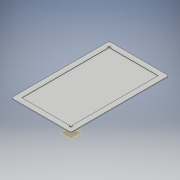
# Autodesk Inventor part: Lid
Saved by Autodesk Inventor 2019 (Build 230136000, 136)
## iProperties
Created: 2018-10-23
Part Number: Lid
Material: Generic
Document SubType Name: Modeling
Designer: Administrator
Density: 1 g/cm^3
Appearance: Default
Author: Administrator
Autodesk Inventor part; units mm, degrees
ref_plane "YZ Plane" through (0, 0, 0) normal (1, 0, 0) x (0, 1, 0)
ref_plane "XZ Plane" through (0, 0, 0) normal (0, 1, 0) x (-1, 0, 0)
ref_plane "XY Plane" through (0, 0, 0) normal (0, 0, 1) x (1, 0, 0)
ref_plane "Work Plane1" through (0, 41.656, 0) normal (0, 1, 0) x (1, 0, 0)
sketch "Sketch2" plane through (0, 41.656, 0) normal (0, 1, 0) x (1, 0, 0)
  line L0 (-118.364, 207.264) -> (-10.414, 207.264) projected
  arc A0 (-4.064, 200.914) -> (-10.414, 207.264) centre (-10.414, 200.914) ccw projected
  line L1 (-4.064, 200.914) -> (-4.064, 10.414) projected
  arc A1 (-10.414, 4.064) -> (-4.064, 10.414) centre (-10.414, 10.414) ccw projected
  line L2 (-10.414, 4.064) -> (-118.364, 4.064) projected
  arc A2 (-124.714, 10.414) -> (-118.364, 4.064) centre (-118.364, 10.414) ccw projected
  line L3 (-124.714, 10.414) -> (-124.714, 200.914) projected
  arc A3 (-118.364, 207.264) -> (-124.714, 200.914) centre (-118.364, 200.914) ccw projected
  line L4 (-128.778, 208.153) -> (-128.778, 3.175) projected
  arc A4 (-128.778, 3.175) -> (-125.603, 0) centre (-125.603, 3.175) ccw projected
  line L5 (-125.603, 0) -> (-3.175, 0) projected
  arc A5 (-3.175, 0) -> (0, 3.175) centre (-3.175, 3.175) ccw projected
  line L6 (0, 3.175) -> (0, 208.153) projected
  arc A6 (0, 208.153) -> (-3.175, 211.328) centre (-3.175, 208.153) ccw projected
  line L7 (-3.175, 211.328) -> (-125.603, 211.328) projected
  arc A7 (-125.603, 211.328) -> (-128.778, 208.153) centre (-125.603, 208.153) ccw projected
  circle A8 centre (-117.348, 199.898) radius 2.794 projected
  circle A9 centre (-11.43, 11.43) radius 2.794 projected
  line L8 (-117.348, 199.898) -> (-11.43, 199.898)
  line L9 (-11.43, 199.898) -> (-11.43, 11.43)
  line L10 (-11.43, 11.43) -> (-117.348, 11.43)
  line L11 (-117.348, 11.43) -> (-117.348, 199.898)
  point P0 (0, 0)
  constraints: 8 end point, 2 parallel, 1 horizontal, 1 perpendicular
extrude "Extrusion5" add sketch "Sketch2" along normal blind 1.27 contours L0 A0 L1 A1 L2 A2 L3 A3 | A7 L7 A6 L6 A5 L5 A4 L4
extrude "Extrusion6" add sketch "Sketch2" along normal blind 0.508 contours L8 L9 A9 L10 L11 A8 | A8 L11 L8 | L9 L10 A9 picked at (-115.5087, 199.6908) picked at (-13.2693, 11.6372)
body "Solid1"
